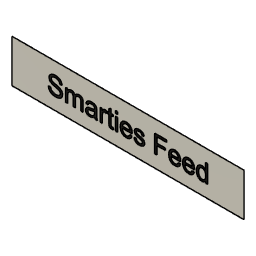
smartie_sorter_3000 (Autodesk Fusion 360 archive; units mm, degrees)
design "Smarties Feed Label"
part number: 2025-04-13-10-05-08-737
Autodesk Fusion 360 part; units mm, degrees
sketch "Sticker" plane through (0, 0, 0) normal (0, 1, 0) x (1, 0, 0)
  line L0 (0, 0) -> (65, 0)
  line L1 (65, 0) -> (65, -12)
  line L2 (65, -12) -> (0, -12)
  line L3 (0, -12) -> (0, 0)
  dimension "d1" = 12
  dimension "d2" = 65
  constraint horizontal L0
  constraint vertical L1
  constraint horizontal L2
  constraint vertical L3
  constraint coincident L0.start L3.end
  measures "d1" distance of L0.end L1.end
  measures "d2" distance of L0.start L0.end
extrude "Extrude1" add sketch "Sticker" along normal blind 0.01 makes body 1
sketch "Text" plane through (0, 0, 0) normal (0, -1, 0) x (1, 0, 0)
  line L0 (65, 12) -> (0, 12)
  line L1 (0, 12) -> (0, 0)
  line L2 (0, 0) -> (65, 0)
  line L3 (65, 0) -> (65, 12)
  line L4 (0, 0) -> (65, 0) construction
  line L5 (65, 0) -> (65, 12) construction
  line L6 (65, 12) -> (0, 12) construction
  line L7 (0, 12) -> (0, 0) construction
  dimension "d5" = 5
  text T0 "Smarties Feed" font "Arial" height 5 align centre middle in box 65 x 12 at (0, 0) x (1, 0) y (0, 1) spacing 1 kerned
  constraint coincident L2.end
  constraint coincident L0.end
extrude "Extrude2" add sketch "Text" along normal blind 0.01 separate body text T0 makes body 2 at (15.2098, 0, 5.3338) makes body 3 at (24.9062, 0, 5.3395) makes body 4 at (29.3878, 0, 8.0293) makes body 5 at (29.3878, 0, 4.7074) makes body 6 at (36.084, 0, 5.3662) makes body 7 at (46.1272, 0, 5.3224) makes body 8 at (50.0119, 0, 5.3224) makes body 9 at (40.1779, 0, 5.9238) makes body 10 at (32.5426, 0, 5.3224) makes body 11 at (54.6076, 0, 5.8807) makes body 12 at (27.554, 0, 5.244) makes body 13 at (23.5463, 0, 4.5282) makes body 14 at (12.6004, 0, 5.8956)
named bodies: "Sticker", "Text 2", "Text 4", "Text 7", "Text 6", "Text 9", "Text 11", "Text 12", "Text 10", "Text 8", "Text 13", "Text 5", "Text 3", "Text 1"

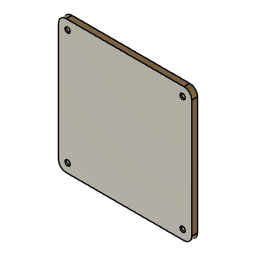
design "Bottom Access Panel"
Autodesk Fusion 360 part; units mm, degrees
sketch "Bottom Access Panel" plane through (0, 0, 0) normal (0, 1, 0) x (1, 0, 0)
  line L0 (0, 0) -> (139, 0)
  line L1 (139, 0) -> (139, -139)
  line L2 (139, -139) -> (0, -139)
  line L3 (0, -139) -> (0, 0)
  dimension "d1" = 139
  dimension "d2" = 139
  constraint horizontal L0
  constraint vertical L1
  constraint horizontal L2
  constraint vertical L3
  constraint coincident L0.start L3.end
  measures "d1" distance of L0.start L0.end
  measures "d2" distance of L0.end L1.end
extrude "Extrude1" add sketch "Bottom Access Panel" along normal blind 6
fillet "Fillet1" radius 8 4 edges at (0, 3, 139) (139, 3, 139) (139, 3, 0) (0, 3, 0)
sketch "Magnet Holes" plane through (0, 0, 0) normal (0, 1, 0) x (1, 0, 0)
  arc A0 (8, 0) -> (0, -8) centre (8, -8) ccw
  line L0 (8, 0) -> (131, 0)
  arc A1 (139, -8) -> (131, 0) centre (131, -8) ccw
  line L1 (139, -8) -> (139, -131)
  arc A2 (131, -139) -> (139, -131) centre (131, -131) ccw
  line L2 (131, -139) -> (8, -139)
  arc A3 (0, -131) -> (8, -139) centre (8, -131) ccw
  line L3 (0, -131) -> (0, -8)
  circle A4 centre (9.5, -129.5) radius 2.75
  circle A5 centre (129.5, -129.5) radius 2.75
  circle A6 centre (9.5, -9.5) radius 2.75
  circle A7 centre (129.5, -9.5) radius 2.75
  dimension "d20" = 5.5
  dimension "d21" = 5.5
  dimension "d22" = 5.5
  dimension "d23" = 5.5
  dimension "d24" = 9.5
  dimension "d25" = 9.5
  dimension "d26" = 9.5
  dimension "d27" = 9.5
  dimension "d28" = 9.5
  dimension "d29" = 9.5
  dimension "d30" = 9.5
  dimension "d31" = 9.5
  measures "d20" diameter of A4
  measures "d21" diameter of A5
  measures "d22" diameter of A6
  measures "d23" diameter of A7
  measures "d24" distance of L1 A5.centre
  measures "d25" distance of L2 A5.centre
  measures "d26" distance of L3 A4.centre
  measures "d27" distance of L2 A4.centre
  measures "d28" distance of L0 A6.centre
  measures "d29" distance of L3 A6.centre
  measures "d30" distance of L1 A7.centre
  measures "d31" distance of L0 A7.centre
extrude "Extrude3" cut sketch "Magnet Holes" along normal blind 1.5 contours A4 | A5 | A6 | A7
equation "mdfThickness = 6 mm" comment "Thickness of the MDF fibre board"
equation "d4 = mdfThickness"
equation "filletRadius = 8 mm" comment "Radius to use for fillets"
equation "d15 = filletRadius"
named bodies: "Bottom Access Panel"

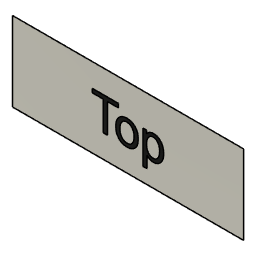
design "Top Label"
part number: 2025-04-13-09-56-45-957
Autodesk Fusion 360 part; units mm, degrees
sketch "Sticker" plane through (0, 0, 0) normal (0, 1, 0) x (1, 0, 0)
  line L0 (0, 0) -> (35, 0)
  line L1 (35, 0) -> (35, -12)
  line L2 (35, -12) -> (0, -12)
  line L3 (0, -12) -> (0, 0)
  dimension "d1" = 35
  dimension "d2" = 12
  constraint horizontal L0
  constraint vertical L1
  constraint horizontal L2
  constraint vertical L3
  constraint coincident L0.start L3.end
  measures "d1" distance of L0.start L0.end
  measures "d2" distance of L0.end L1.end
extrude "Extrude1" add sketch "Sticker" along normal blind 0.01 makes body 1
sketch "Text" plane through (0, 0, 0) normal (0, -1, 0) x (1, 0, 0)
  line L0 (35, 12) -> (0, 12)
  line L1 (0, 12) -> (0, 0)
  line L2 (0, 0) -> (35, 0)
  line L3 (35, 0) -> (35, 12)
  line L4 (0, 0) -> (35, 0) construction
  line L5 (35, 0) -> (35, 12) construction
  line L6 (35, 12) -> (0, 12) construction
  line L7 (0, 12) -> (0, 0) construction
  dimension "d5" = 5
  text T0 "Top" font "Arial" height 5 align centre middle in box 35 x 12 at (0, 0) x (1, 0) y (0, 1) spacing 1 kerned
  constraint coincident L2.end
  constraint coincident L0.end
extrude "Extrude2" add sketch "Text" along normal blind 0.01 separate body text T0 makes body 2 at (19.9566, 0, 4.7193) makes body 3 at (15.8803, 0, 5.5613) makes body 4 at (14.1792, 0, 4.97)
named bodies: "Sticker", "Text 3", "Text 2", "Text 1"
